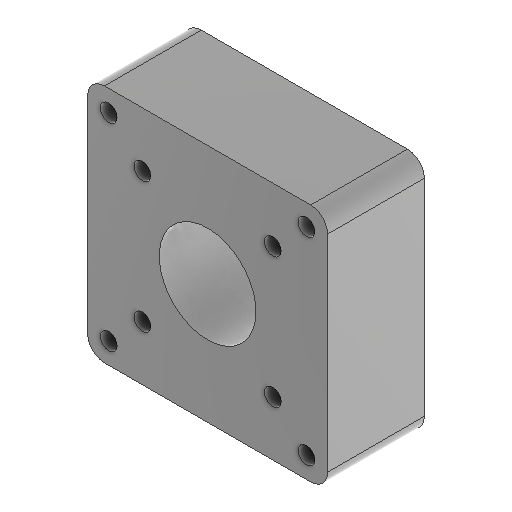
# Autodesk Inventor part: 00_NEMA17_Perestalticpump_Adapter
Saved by Autodesk Inventor 2024.1 (Build 281209000, 209)
## iProperties
Created: 2024-03-02
Part Number: 00_NEMA17_Perestalticpump_Adapter
Material: Generisch
Document SubType Name: Modeling
Designer: diederichbenedict
Density: 1 g/cm^3
Appearance: Glatt - Mittelgrau
Vendor: Amazon
Mass: 62.543 g
Surface Area: 144.987 cm^2
Volume: 62.543 cm^3
Author: diederichbenedict
Autodesk Inventor part; units mm, degrees
ref_plane "YZ Plane" through (0, 0, 0) normal (1, 0, 0) x (0, 1, 0)
ref_plane "XZ Plane" through (0, 0, 0) normal (0, 1, 0) x (-1, 0, 0)
ref_plane "XY Plane" through (0, 0, 0) normal (0, 0, 1) x (1, 0, 0)
ref_plane "Arbeitsebene1" through (63.727, -21.9316, 9.2792) normal (0, -1, 0) x (1, 0, 0)
sketch "Skizze1" plane through (63.727, -21.9316, 9.2792) normal (0, -1, 0) x (1, 0, 0)
  line L0 (-20.15, -16.7358) -> (-16.7358, -20.15) projected
  line L1 (-16.7358, -20.15) -> (16.7358, -20.15) projected
  line L2 (16.7358, -20.15) -> (20.15, -16.7358) projected
  line L3 (20.15, -16.7358) -> (20.15, 16.7358) projected
  line L4 (20.15, 16.7358) -> (16.7358, 20.15) projected
  line L5 (16.7358, 20.15) -> (-16.7358, 20.15) projected
  line L6 (-16.7358, 20.15) -> (-20.15, 16.7358) projected
  line L7 (-20.15, 16.7358) -> (-20.15, -16.7358) projected
  circle A0 centre (-15.5, -15.5) radius 2 projected
  circle A1 centre (15.5, -15.5) radius 2 projected
  circle A2 centre (15.5, 15.5) radius 2 projected
  circle A3 centre (-15.5, 15.5) radius 2 projected
  circle A4 centre (0, 0) radius 11.5 projected
  line L8 (24.5, -28.5) -> (-24.5, -28.5)
  line L9 (-28.5, -24.5) -> (-28.5, 24.5)
  line L10 (-24.5, 28.5) -> (24.5, 28.5)
  line L11 (28.5, 24.5) -> (28.5, -24.5)
  line L12 (28.5, -28.5) -> (-28.5, 28.5) construction
  line L13 (-28.5, -28.5) -> (28.5, 28.5) construction
  arc A5 (-24.5, 28.5) -> (-28.5, 24.5) centre (-24.5, 24.5) ccw
  arc A6 (28.5, 24.5) -> (24.5, 28.5) centre (24.5, 24.5) ccw
  arc A7 (24.5, -28.5) -> (28.5, -24.5) centre (24.5, -24.5) ccw
  arc A8 (-28.5, -24.5) -> (-24.5, -28.5) centre (-24.5, -24.5) ccw
  line L14 (23.5, -23.5) -> (-23.5, -23.5) construction
  line L15 (-23.5, -23.5) -> (-23.5, 23.5) construction
  line L16 (-23.5, 23.5) -> (23.5, 23.5) construction
  line L17 (23.5, 23.5) -> (23.5, -23.5) construction
  line L18 (23.5, -23.5) -> (-23.5, 23.5) construction
  line L19 (-23.5, -23.5) -> (23.5, 23.5) construction
  circle A9 centre (-23.5, 23.5) radius 2
  circle A10 centre (23.5, 23.5) radius 2
  circle A11 centre (23.5, -23.5) radius 2
  circle A12 centre (-23.5, -23.5) radius 2
  point P0 (-63.727, -9.2792)
  dimension "d0" = 57
  dimension "d1" = 57
  dimension "d2" = 4
  dimension "d3" = 47
  dimension "d4" = 47
  dimension "d5" = 4
  dimension "d6" = 4
  dimension "d7" = 4
  dimension "d8" = 4
  constraints: 24 end point, 10 point on line, 8 centre point, 8 point on circle, 8 tangent, 4 midpoint, 4 parallel, 3 coincident, 3 equal radius, 2 horizontal, 2 perpendicular
  measures "d0" distance of L12.end L13.end
  measures "d1" distance of L13.start L12.end
  measures "d2" radius of A5
  measures "d3" distance of L15.end L16.end
  measures "d4" distance of L14.end L15.end
  measures "d5" diameter of A9
  measures "d6" diameter of A10
  measures "d7" diameter of A11
  measures "d8" diameter of A12
extrude "Extrusion1" add sketch "Skizze1" along normal blind 23 contours L7 L6 L5 L4 L3 L2 L1 L0 | L8 A8 L9 A5 L10 A6 L11 A7
